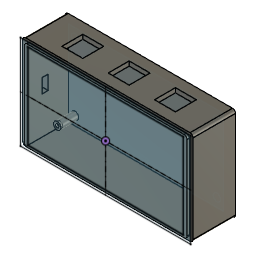
ESP32 Alarm Clock_ (Autodesk Fusion 360 archive; units mm, degrees)
design "Wecker Case Hinten redesign"
part number: 2026-04-11-20-32-26-952
Autodesk Fusion 360 part; units mm, degrees
derive "Abgeleiteter Kontext1"
sketch "Skizze1" plane through (0, 0, 0) normal (0, 1, 0) x (1, 0, 0)
  line L0 (-57, 31.5) -> (57, 31.5)
  line L1 (57, 31.5) -> (57, -31.5)
  line L2 (57, -31.5) -> (-57, -31.5)
  line L3 (-57, -31.5) -> (-57, 31.5)
  line L4 (0, -31.5) -> (0, 31.5) construction
  line L5 (57, 0) -> (-57, 0) construction
  dimension "d1" = 114
  dimension "d2" = 63
  constraint horizontal L0
  constraint vertical L1
  constraint horizontal L2
  constraint vertical L3
  constraint midpoint L2 L4.start
  constraint midpoint L0 L4.end
  constraint midpoint L1 L5.start
  constraint midpoint L3 L5.end
  constraint coincident origin L5
  constraint coincident origin L4
  measures "d1" distance of L0.start L0.end
  measures "d2" distance of L0.start L2.end
extrude "Extrusion1" add sketch "Skizze1" along normal blind 30
sketch "Skizze2" plane through (0, 0, 0) normal (0, -1, 0) x (1, 0, 0)
  line L0 (57, 31.5) -> (-57, 31.5)
  line L1 (-57, 31.5) -> (-57, -31.5)
  line L2 (-57, -31.5) -> (57, -31.5)
  line L3 (57, -31.5) -> (57, 31.5)
  line L4 (-52, 28.5) -> (52, 28.5)
  line L5 (52, 28.5) -> (52, -28.5)
  line L6 (52, -28.5) -> (-52, -28.5)
  line L7 (-52, -28.5) -> (-52, 28.5)
  line L8 (0, 28.5) -> (0, -28.5) construction
  line L9 (52, 0) -> (-52, 0) construction
  dimension "d5" = 104
  dimension "d6" = 57
  constraint horizontal L4
  constraint vertical L5
  constraint horizontal L6
  constraint vertical L7
  constraint midpoint L4 L8.start
  constraint midpoint L6 L8.end
  constraint midpoint L5 L9.start
  constraint midpoint L7 L9.end
  constraint coincident origin L8
  constraint coincident origin L9
  measures "d5" distance of L4.start L4.end
  measures "d6" distance of L4.start L6.end
extrude "Extrusion2" cut sketch "Skizze2" against normal blind 27 contours L4 L5 L6 L7
sketch "Skizze3" plane through (0, 0, 0) normal (0, -1, 0) x (1, 0, 0)
  line L0 (52, 28.5) -> (52, -28.5)
  line L1 (52, -28.5) -> (-52, -28.5)
  line L2 (-52, -28.5) -> (-52, 28.5)
  line L3 (-52, 28.5) -> (52, 28.5)
  line L4 (57, 31.5) -> (-57, 31.5)
  line L5 (-57, 31.5) -> (-57, -31.5)
  line L6 (-57, -31.5) -> (57, -31.5)
  line L7 (57, -31.5) -> (57, 31.5)
  line L8 (-54.5, 30) -> (54.5, 30)
  line L9 (54.5, 30) -> (54.5, -30)
  line L10 (54.5, -30) -> (-54.5, -30)
  line L11 (-54.5, -30) -> (-54.5, 30)
  line L12 (0, 30) -> (0, -30) construction
  line L13 (54.5, 0) -> (-54.5, 0) construction
  line L14 (57, 31.5) -> (-57, 31.5)
  line L15 (-57, 31.5) -> (-57, -31.5)
  line L16 (57, -31.5) -> (57, 31.5)
  line L17 (-57, -31.5) -> (57, -31.5)
  line L18 (-52, -28.5) -> (-52, 28.5)
  line L19 (52, -28.5) -> (-52, -28.5)
  line L20 (57, 31.5) -> (-57, 31.5)
  dimension "d9" = 109
  dimension "d10" = 60
  dimension "d97" = 2.5
  dimension "d98" = 2.5
  dimension "d99" = 1.5
  dimension "d100" = 1.5
  dimension "d101" = 2.5
  dimension "d125" = 1.5
  constraint horizontal L8
  constraint vertical L9
  constraint horizontal L10
  constraint vertical L11
  constraint midpoint L8 L12.start
  constraint midpoint L10 L12.end
  constraint midpoint L9 L13.start
  constraint midpoint L11 L13.end
  constraint coincident origin L12
  constraint coincident origin L13
  measures "d9" distance of L8.start L8.end
  measures "d10" distance of L8.start L10.end
  measures "d97" distance of L11 L15
  measures "d98" distance of L11 L18
  measures "d99" distance of L10 L19
  measures "d100" distance of L6 L10
  measures "d101" distance of L9 L16
  measures "d125" distance of L8 L20
extrude "Extrusion3" cut sketch "Skizze3" against normal blind 1.5 contours L4 L5 L6 L7 L14 L15 L16 L17 L20
sketch "Skizze4" plane through (0, 30, 0) normal (0, 1, 0) x (-1, 0, 0)
  line L0 (57, 31.5) -> (-57, 31.5)
  line L1 (-57, 31.5) -> (-57, -31.5)
  line L2 (-57, -31.5) -> (57, -31.5)
  line L3 (57, -31.5) -> (57, 31.5)
  line L4 (0, 31.5) -> (0, -31.5) construction
  line L5 (-57, 0) -> (57, 0) construction
  point P0 (-47.5, 23.5)
  point P1 (47.5, 23.5)
  point P2 (-47.5, -23.5)
  point P3 (47.5, -23.5)
  dimension "d13" = 9.5
  dimension "d14" = 8
  constraint midpoint L0 L4.start
  constraint midpoint L2 L4.end
  constraint midpoint L1 L5.start
  constraint midpoint L3 L5.end
  constraint symmetric L4 P0 P1
  constraint symmetric L5 P0 P2
  constraint symmetric L5 P1 P3
  measures "d13" distance of L1 P0
  measures "d14" distance of L0 P0
sketch "Skizze5" plane through (0, 27, 0) normal (0, -1, 0) x (1, 0, 0)
  line L0 (-52, -28.5) -> (52, -28.5)
  line L1 (52, -28.5) -> (52, 28.5)
  line L2 (52, 28.5) -> (-52, 28.5)
  line L3 (-52, 28.5) -> (-52, -28.5)
  circle A0 centre (-47.5, 22.5) radius 2.5
  line L4 (0, 28.5) -> (0, -28) construction
  line L5 (52, 0) -> (-52, 0) construction
  circle A1 centre (47.5, 22.5) radius 2.5
  circle A2 centre (-47.5, -22.5) radius 2.5
  circle A3 centre (47.5, -22.5) radius 2.5
  line L6 (-57, -31.5) -> (-57, 31.5)
  point P0 (-47.5, 23.5)
  point P1 (47.5, 23.5)
  point P2 (-47.5, -23.5)
  point P3 (47.5, -23.5)
  dimension "d15" = 5
  dimension "d90" = 6
  dimension "d91" = 4.5
  constraint midpoint L2 L4.start
  constraint perpendicular L2 L4
  constraint midpoint L1 L5.start
  constraint midpoint L3 L5.end
  constraint symmetric A0 L4 A1
  constraint symmetric A0 L5 A2
  constraint symmetric L5 A1 A3
  measures "d15" diameter of A0
  measures "d90" distance of L2 A0.centre
  measures "d91" distance of L3 A0.centre
extrude "Extrusion4" add sketch "Skizze5" along normal blind 11.9 contours A0 | A1 | A2 | A3
fillet "Abrundung1" radius 2 8 edges at (-57, 15.75, 31.5) (-54.5, 0.75, 30) (-54.5, 0.75, -30) (-57, 15.75, -31.5) (57, 15.75, -31.5) (54.5, 0.75, -30) (57, 15.75, 31.5) (54.5, 0.75, 30)
sketch "Skizze14" plane through (0, 30, 0) normal (0, 1, 0) x (-1, 0, 0)
  arc A0 (-55, 31.5) -> (-57, 29.5) centre (-55, 29.5) ccw
  line L0 (-57, 29.5) -> (-57, -29.5)
  arc A1 (-57, -29.5) -> (-55, -31.5) centre (-55, -29.5) ccw
  line L1 (-55, -31.5) -> (55, -31.5)
  arc A2 (55, -31.5) -> (57, -29.5) centre (55, -29.5) ccw
  line L2 (57, -29.5) -> (57, 29.5)
  arc A3 (57, 29.5) -> (55, 31.5) centre (55, 29.5) ccw
  line L3 (55, 31.5) -> (-55, 31.5)
  circle A4 centre (-47.5, 22.5) radius 2.5
  circle A5 centre (47.5, 22.5) radius 2.5
  circle A6 centre (47.5, -22.5) radius 2.5
  circle A7 centre (-47.5, -22.5) radius 2.5
sketch "Skizze15" plane through (0, 27, 0) normal (0, -1, 0) x (1, 0, 0)
  circle A0 centre (-47.5, -22.5) radius 2.5
  circle A1 centre (-47.5, 22.5) radius 2.5
  circle A2 centre (47.5, -22.5) radius 2.5
  circle A3 centre (47.5, 22.5) radius 2.5
  line L0 (-52, -28.5) -> (52, -28.5)
  line L1 (52, -28.5) -> (52, 28.5)
  line L2 (52, 28.5) -> (-52, 28.5)
  line L3 (-52, 28.5) -> (-52, -28.5)
hole "Bohrung6" at (47.5, 30, 22.5) at (-47.5, 30, 22.5) at (-47.5, 30, -22.5) at (47.5, 30, -22.5) direction (0, -1, 0) diameter 2.3 depth 16.5 tip angle 118 counterbore diameter 4.3 counterbore depth 13.5
sketch "Skizze16" plane through (0, 0, 31.5) normal (0, 0, 1) x (-1, 0, 0)
  line L0 (-55, -1.5) -> (-55, -30)
  line L1 (-55, -30) -> (55, -30)
  line L2 (55, -30) -> (55, -1.5)
  line L3 (55, -1.5) -> (-55, -1.5)
  line L4 (38, -22.75) -> (24, -22.75)
  line L5 (24, -22.75) -> (24, -8.75)
  line L6 (24, -8.75) -> (38, -8.75)
  line L7 (38, -8.75) -> (38, -22.75)
  line L8 (7, -22.75) -> (-7, -22.75)
  line L9 (-7, -22.75) -> (-7, -8.75)
  line L10 (-7, -8.75) -> (7, -8.75)
  line L11 (7, -8.75) -> (7, -22.75)
  line L12 (55, -30) -> (-55, -30)
  line L13 (-24, -22.75) -> (-38, -22.75)
  line L14 (-38, -22.75) -> (-38, -8.75)
  line L15 (-38, -8.75) -> (-24, -8.75)
  line L16 (-24, -8.75) -> (-24, -22.75)
  dimension "d102" = 110
  dimension "d103" = 28.5
  dimension "d104" = 14
  dimension "d105" = 14
  dimension "d106" = 17
  dimension "d107" = 7.25
  dimension "d114" = 14
  dimension "d115" = 14
  dimension "d116" = 7.25
  dimension "d117" = 48
  dimension "d118" = 14
  dimension "d119" = 14
  dimension "d120" = 7.25
  dimension "d121" = 79
  dimension "d122" = 17
  dimension "d126" = 110
  constraint horizontal L4
  constraint vertical L5
  constraint horizontal L6
  constraint vertical L7
  constraint horizontal L8
  constraint vertical L9
  constraint horizontal L10
  constraint vertical L11
  constraint horizontal L13
  constraint vertical L14
  constraint horizontal L15
  constraint vertical L16
  measures "d102" distance of L0 L2
  measures "d103" distance of L1 L3
  measures "d104" distance of L4.start L4.end
  measures "d105" distance of L4.start L6.end
  measures "d106" distance of L2 L7
  measures "d107" distance of L1 L4
  measures "d114" distance of L8.start L8.end
  measures "d115" distance of L8.start L10.end
  measures "d116" distance of L8 L12
  measures "d117" distance of L2 L11
  measures "d118" distance of L13.start L13.end
  measures "d119" distance of L13.start L15.end
  measures "d120" distance of L1 L13
  measures "d121" distance of L2 L16
  measures "d122" distance of L0 L14
  measures "d126" distance of L0 L2
extrude "Extrusion12" cut sketch "Skizze16" against normal blind 4 contours L4 L5 L6 L7 | L8 L9 L10 L11 | L13 L14 L15 L16
sketch "Skizze17" plane through (-57, 0, 0) normal (-1, 0, 0) x (0, -1, 0)
  line L0 (-30, -29.5) -> (-1.5, -29.5)
  line L1 (-1.5, -29.5) -> (-1.5, 29.5)
  line L2 (-1.5, 29.5) -> (-30, 29.5)
  line L3 (-30, 29.5) -> (-30, -29.5)
  line L4 (0, 28.5) -> (-27, 28.5)
  line L5 (-27, 28.5) -> (-27, -28.5)
  line L6 (0, -28.5) -> (-27, -28.5)
  line L7 (-13.5, 6) -> (-9.5, 6)
  line L8 (-9.5, 6) -> (-9.5, -3.5)
  line L9 (-9.5, -3.5) -> (-13.5, -3.5)
  line L10 (-13.5, -3.5) -> (-13.5, 6)
  dimension "d127" = 59
  dimension "d128" = 4
  dimension "d129" = 9.5
  dimension "d130" = 13.5
  dimension "d131" = 22.5
  constraint horizontal L7
  constraint vertical L8
  constraint horizontal L9
  constraint vertical L10
  measures "d127" distance of L0 L2
  measures "d128" distance of L7.start L7.end
  measures "d129" distance of L7.start L9.end
  measures "d130" distance of L5 L10
  measures "d131" distance of L4 L7
extrude "Extrusion13" cut sketch "Skizze17" against normal blind 6 contours L7 L8 L9 L10
